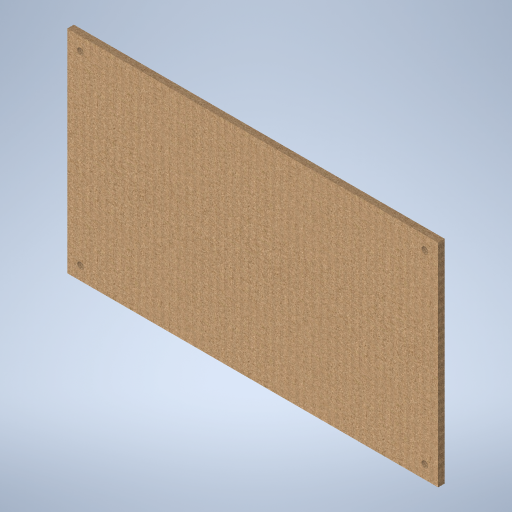
# Autodesk Inventor part: BasePiso
Saved by Autodesk Inventor 2023.1 (Build 271208000, 208)
## iProperties
Created: 2022-11-01
Part Number: BasePiso
Material: MDF Medium Density Fiberboard
Document SubType Name: Modeling
Designer: Daniel Peña
Density: 0.8 g/cm^3
Appearance: Cardboard - Corrugated
Author: Daniel Peña
Autodesk Inventor part; units mm, degrees
ref_plane "YZ Plane" through (0, 0, 0) normal (1, 0, 0) x (0, 1, 0)
ref_plane "XZ Plane" through (0, 0, 0) normal (0, 1, 0) x (-1, 0, 0)
ref_plane "XY Plane" through (0, 0, 0) normal (0, 0, 1) x (1, 0, 0)
sketch "Sketch1" plane through (0, 0, 0) normal (0, 0, 1) x (1, 0, 0)
  line L0 (-140, -80) -> (140, -80)
  line L1 (140, -80) -> (140, 80)
  line L2 (140, 80) -> (-140, 80)
  line L3 (-140, 80) -> (-140, -80)
  point P0 (0, 0)
  constraints: 8 end point, 2 parallel, 1 horizontal, 1 perpendicular
extrude "Extrusion1" add sketch "Sketch1" along normal blind 5
sketch "Sketch2" plane through (0, 0, 5) normal (0, 0, 1) x (1, 0, 0)
  line L0 (0, -70.9662) -> (0, 58.0253) construction
  line L1 (62.9304, 0) -> (-65.435, 0) construction
  line L2 (140, -80) -> (140, 80) construction
  line L3 (-140, -80) -> (140, -80) construction
  point P0 (0, 0)
  point P1 (130, -70)
  point P2 (130, 70)
  point P3 (-130, 70)
  point P4 (-130, -70)
  dimension "d2" = 10
  dimension "d3" = 10
  constraints: 4 end point, 4 symmetric about line, 1 horizontal, 1 vertical
  measures "d2" distance from line of L2 point (130, -70)
  measures "d3" distance from line of L3 point (130, -70)
hole "Hole1" at (130, -70, 5) at (130, 70, 5) at (-130, 70, 5) at (-130, -70, 5) direction (0, 0, -1) diameter 5 end through all
body "Solid1"
